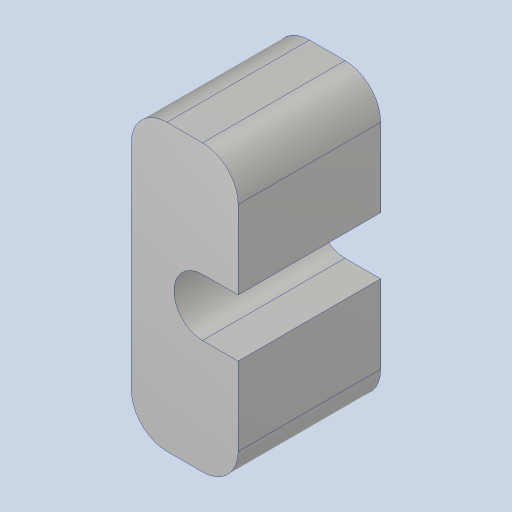
# Autodesk Inventor part: CANdle spacer
Saved by Autodesk Inventor 2023.4 (Build 274418000, 418)
## iProperties
Created: 2025-02-12
Part Number: CANdle spacer
Material: Aluminum 6061
Document SubType Name: Modeling
Designer: mavericks
Density: 2.7 g/cm^3
Appearance: Aluminum - Flat
Author: mavericks
Autodesk Inventor part; units mm, degrees
ref_plane "YZ Plane" through (0, 0, 0) normal (1, 0, 0) x (0, 1, 0)
ref_plane "XZ Plane" through (0, 0, 0) normal (0, 1, 0) x (-1, 0, 0)
ref_plane "XY Plane" through (0, 0, 0) normal (0, 0, 1) x (1, 0, 0)
sketch "Sketch1" plane through (0, 0, 0) normal (0, 0, 1) x (1, 0, 0)
  line L0 (-4.7625, 12.7) -> (4.7625, 12.7)
  line L1 (4.7625, 12.7) -> (4.7625, -12.7)
  line L2 (4.7625, -12.7) -> (-4.7625, -12.7)
  line L3 (-4.7625, -12.7) -> (-4.7625, 12.7)
  line L4 (-4.7625, 12.7) -> (4.7625, -12.7) construction
  line L5 (4.7625, 12.7) -> (-4.7625, -12.7) construction
  circle A0 centre (1.5875, 0) radius 2.5527
  line L6 (1.5875, 2.5527) -> (4.7625, 2.5527)
  line L7 (1.5875, -2.5527) -> (4.7625, -2.5527)
  point P0 (0, 0)
  dimension "d0" = 9.525
  dimension "d1" = 25.4
  dimension "d2" = 3.175
  dimension "d3" = 12.7
  dimension "d4" = 5.1054
  constraints: 16 end point, 3 perpendicular, 2 midpoint, 2 parallel, 2 point on circle, 2 point on line, 2 tangent, 1 centre point, 1 coincident, 1 horizontal
  measures "d0" distance of L1.end L2.end
  measures "d1" distance of L0.end L1.end
  measures "d2" distance from line of L1 point (1.587, 0)
  measures "d3" distance from line of L0 point (1.587, 0)
  measures "d4" diameter of A0
extrude "Extrusion1" add sketch "Sketch1" along normal blind 12.7 contours L0 L1 L6 A0 L7 L2 L3
fillet "Fillet1" radius 3.175 4 edges at (-4.7625, 12.7, 6.35) (4.7625, 12.7, 6.35) (4.7625, -12.7, 6.35) (-4.7625, -12.7, 6.35)
body "Solid1"
